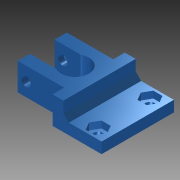
# Autodesk Inventor part: ZAxisEndstopMount
Saved by Autodesk Inventor 2015 SP1 (Build 190203100, 203)
## iProperties
Created: 2015-01-30
Part Number: ZAxisEndstopMount
Material: Generic
Document SubType Name: Modeling
Designer: Jack
Density: 1 g/cm^3
Appearance: Cyan
Author: Jack
Autodesk Inventor part; units mm, degrees
ref_plane "YZ Plane" through (0, 0, 0) normal (1, 0, 0) x (0, 1, 0)
ref_plane "XZ Plane" through (0, 0, 0) normal (0, 1, 0) x (-1, 0, 0)
ref_plane "XY Plane" through (0, 0, 0) normal (0, 0, 1) x (1, 0, 0)
sketch "Sketch1" plane through (0, 0, 0) normal (0, 0, 1) x (1, 0, 0)
  arc A0 (-2.4, -4.5) -> (-2.4, 4.5) centre (0, 0) ccw
  line L0 (-2.4, 4.5) -> (-12, 4.5)
  line L1 (-12, 4.5) -> (-12, 9)
  line L2 (-12, 9) -> (5, 9)
  line L3 (5, -9) -> (-12, -9)
  line L4 (-12, -9) -> (-12, -4.5)
  line L5 (-12, -4.5) -> (-2.4, -4.5)
  line L6 (5, 9) -> (5, 13.25)
  line L7 (5, -9) -> (5, -13.25)
  line L8 (5, 13.25) -> (9, 13.25)
  line L9 (9, 13.25) -> (9, -13.25)
  line L10 (9, -13.25) -> (5, -13.25)
  dimension "d0" = 10.2
  dimension "d1" = 9
  dimension "d2" = 12
  dimension "d3" = 9
  dimension "d7" = 26.5
  dimension "d8" = 4.25
  dimension "d9" = 4
  dimension "d10" = 5
  constraints: 22 end point, 6 perpendicular, 2 equal length, 2 horizontal, 2 point on circle, 2 point on line, 2 vertical, 1 centre point, 1 coincident, 1 vertical alignment
  measures "d0" diameter of A0
  measures "d1" distance from line of point (0, 0) L3
  measures "d2" distance from line of point (0, 0) L4
  measures "d3" distance between parallel lines of L5 L0
  measures "d7" distance of L8.end L9.end
  measures "d8" distance between parallel lines of L2 L8
  measures "d9" distance of L6.end L8.end
  measures "d10" distance from line of point (0, 0) L6
extrude "Extrusion1" add sketch "Sketch1" along normal blind 10
sketch "Sketch4" plane through (5, 13.25, 0) normal (0, 1, 0) x (1, 0, 0)
  line L0 (4, 0) -> (0, 0) projected
  line L1 (4, 0) -> (4, -10) projected
  line L2 (4, 0) -> (4, -10) projected
  line L3 (4, 0) -> (18, 0)
  line L4 (18, 0) -> (18, -4)
  line L5 (18, -4) -> (4, -4)
  point P0 (-5, 0)
  dimension "d22" = 14
  dimension "d24" = 4
  constraints: 6 end point, 2 perpendicular, 2 point on line, 1 collinear, 1 horizontal
  measures "d22" distance of L3.start L3.end
  measures "d24" distance of L3.end L4.end
extrude "Extrusion4" add sketch "Sketch4" against normal up to surface (26.5 mm away)
sketch "Sketch5" plane through (9, 13.25, 4) normal (0, 0, 1) x (1, 0, 0)
  line L0 (0, -26.5) -> (14, -26.5) projected
  line L1 (14, 0) -> (14, -26.5) projected
  line L2 (0, 0) -> (14, 0) projected
  circle A0 centre (9, -3.75) radius 1.75
  circle A1 centre (9, -22.75) radius 1.75
  point P0 (-9, -13.25)
  dimension "d27" = 3.5
  dimension "d28" = 3.75
  dimension "d29" = 3.75
  dimension "d30" = 5
  constraints: 2 centre point, 1 equal radius, 1 vertical alignment
  measures "d27" diameter of A0
  measures "d28" distance from line of L2 A0.centre
  measures "d29" distance from line of L0 A1.centre
  measures "d30" distance from line of L1 A0.centre
extrude "Extrusion5" cut sketch "Sketch5" against normal up to next
sketch "Sketch6" plane through (-12, -9, 0) normal (0, -1, 0) x (1, 0, 0)
  line L0 (0, 10) -> (17, 10) projected
  line L1 (0, 0) -> (0, 10) projected
  circle A0 centre (3, 5) radius 1.75
  point P0 (12, 0)
  dimension "d33" = 3.5
  dimension "d34" = 3
  dimension "d35" = 5
  constraints: 1 centre point
  measures "d33" diameter of A0
  measures "d34" distance from line of L1 A0.centre
  measures "d35" distance from line of L0 A0.centre
extrude "Extrusion6" cut sketch "Sketch6" against normal up to surface (18 mm away)
sketch "Sketch7" plane through (-12, 9, 0) normal (0, 1, 0) x (1, 0, 0)
  circle A0 centre (3, -5) radius 1.75 projected
  line L0 (3, -8.3486) -> (0.1, -6.6743)
  line L1 (0.1, -6.6743) -> (0.1, -3.3257)
  line L2 (0.1, -3.3257) -> (3, -1.6514)
  line L3 (3, -1.6514) -> (5.9, -3.3257)
  line L4 (5.9, -3.3257) -> (5.9, -6.6743)
  line L5 (5.9, -6.6743) -> (3, -8.3486)
  point P0 (12, 0)
  dimension "d38" = 5.8
  constraints: 12 end point, 1 coincident, 1 vertical, 13 other
  measures "d38" distance between parallel lines of L1 L4
extrude "Extrusion7" cut sketch "Sketch7" against normal blind 2.5
sketch "Sketch8" plane through (9, 13.25, 4) normal (0, 0, 1) x (1, 0, 0)
  circle A0 centre (9, -3.75) radius 1.75 projected
  circle A1 centre (9, -22.75) radius 1.75 projected
  line L0 (5.6514, -22.75) -> (7.3257, -19.85)
  line L1 (7.3257, -19.85) -> (10.6743, -19.85)
  line L2 (10.6743, -19.85) -> (12.3486, -22.75)
  line L3 (12.3486, -22.75) -> (10.6743, -25.65)
  line L4 (10.6743, -25.65) -> (7.3257, -25.65)
  line L5 (7.3257, -25.65) -> (5.6514, -22.75)
  line L6 (5.6514, -3.75) -> (7.3257, -0.85)
  line L7 (7.3257, -0.85) -> (10.6743, -0.85)
  line L8 (10.6743, -0.85) -> (12.3486, -3.75)
  line L9 (12.3486, -3.75) -> (10.6743, -6.65)
  line L10 (10.6743, -6.65) -> (7.3257, -6.65)
  line L11 (7.3257, -6.65) -> (5.6514, -3.75)
  point P0 (-9, -13.25)
  dimension "d41" = 5.8
  constraints: 24 end point, 2 coincident, 2 horizontal, 1 parallel, 26 other
  measures "d41" distance between parallel lines of L4 L1
extrude "Extrusion8" cut sketch "Sketch8" against normal blind 2.5
chamfer "Chamfer1" distance 2 angle 45 1 edges at (9, 0, 4)
body "Solid1"
